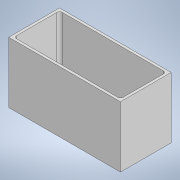
# Autodesk Inventor part: balde
Saved by Autodesk Inventor 2020 (Build 240168000, 168)
## iProperties
Created: 2021-03-20
Part Number: balde
Material: Generic
Document SubType Name: Modeling
Designer: super
Density: 1 g/cm^3
Appearance: Default
Mass: 468.968 g
Surface Area: 1888.13 cm^2
Volume: 468.968 cm^3
Author: super
Autodesk Inventor part; units mm, degrees
ref_plane "YZ Plane" through (0, 0, 0) normal (1, 0, 0) x (0, 1, 0)
ref_plane "XZ Plane" through (0, 0, 0) normal (0, 1, 0) x (-1, 0, 0)
ref_plane "XY Plane" through (0, 0, 0) normal (0, 0, 1) x (1, 0, 0)
sketch "Sketch1" plane through (0, 0, 0) normal (0, 1, 0) x (-1, 0, 0)
  line L0 (0, 0) -> (220, 0)
  line L1 (220, 0) -> (220, -100)
  line L2 (220, -100) -> (0, -100)
  line L3 (0, -100) -> (0, 0)
  dimension "d0" = 220
  dimension "d1" = 100
  constraints: 8 end point, 3 perpendicular, 1 horizontal
  measures "d0" distance of L0.start L0.end
  measures "d1" distance of L2.end L0.start
extrude "Extrusion1" add sketch "Sketch1" along normal blind 120
sketch "Sketch2" plane through (0, 120, 0) normal (0, 1, 0) x (1, 0, 0)
  line L0 (-210, 5) -> (-10, 5)
  line L1 (-5, 10) -> (-5, 90)
  line L2 (-10, 95) -> (-210, 95)
  line L3 (-215, 90) -> (-215, 10)
  line L4 (-220, 100) -> (-220, 0) projected
  line L5 (0, 0) -> (0, 100) projected
  arc A0 (-210, 95) -> (-215, 90) centre (-210, 90) ccw
  arc A1 (-5, 90) -> (-10, 95) centre (-10, 90) ccw
  arc A2 (-10, 5) -> (-5, 10) centre (-10, 10) ccw
  arc A3 (-215, 10) -> (-210, 5) centre (-210, 10) ccw
  point P0 (-215, 5)
  point P1 (-5, 95)
  point P2 (-5, 5)
  point P3 (-215, 95)
  dimension "d4" = 5
  dimension "d5" = 5
  dimension "d6" = 5
  dimension "d7" = 5
  dimension "d8" = 5
  constraints: 8 end point, 8 point on circle, 8 point on line, 8 tangent, 4 centre point, 3 equal radius, 2 parallel, 1 horizontal, 1 perpendicular
  measures "d4" distance from line of L4 point (-215, 5)
  measures "d5" horizontal distance of L5.start point (-5, 5)
  measures "d6" horizontal distance of L4.start point (-215, 95)
  measures "d7" distance from line of L5 point (-5, 95)
  measures "d8" radius of A0
extrude "Extrusion2" cut sketch "Sketch2" against normal blind 115
body "Solid1"
